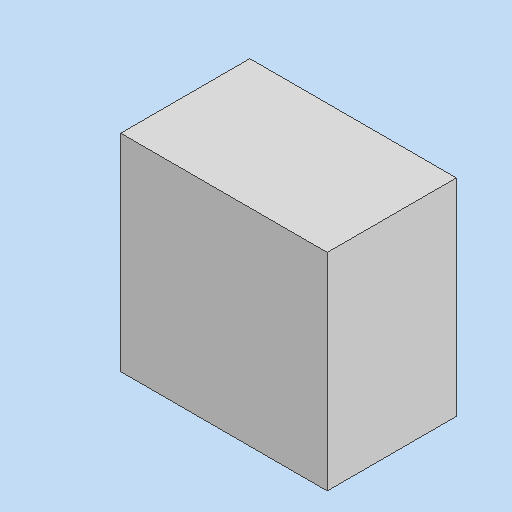
# Autodesk Inventor part: NurdShooterStandin
Saved by Autodesk Inventor 2024.2 (Build 282272000, 272)
## iProperties
Created: 2024-02-06
Part Number: NurdShooterStandin
Material: Generic
Document SubType Name: Modeling
Designer: webbgamers
Density: 1 g/cm^3
Appearance: Default
Author: webbgamers
Autodesk Inventor part; units mm, degrees
ref_plane "YZ Plane" through (0, 0, 0) normal (1, 0, 0) x (0, 1, 0)
ref_plane "XZ Plane" through (0, 0, 0) normal (0, 1, 0) x (-1, 0, 0)
ref_plane "XY Plane" through (0, 0, 0) normal (0, 0, 1) x (1, 0, 0)
ref_plane "Work Plane1" through (1.9437, -39.5479, 0) normal (0, 0, 1) x (1, 0, 0)
sketch "Sketch1" plane through (1.9437, -39.5479, 0) normal (0, 0, 1) x (1, 0, 0)
  line L0 (516.6956, 198.2733) -> (110.2956, 198.2733)
  line L1 (110.2956, 198.2733) -> (110.2956, -208.1267)
  line L2 (110.2956, -208.1267) -> (516.6956, -208.1267)
  line L3 (516.6956, -208.1267) -> (516.6956, 198.2733)
  point P0 (-1.9437, 39.5479)
  dimension "d0" = 406.4
  dimension "d1" = 406.4
  constraints: 8 end point, 2 parallel, 1 horizontal, 1 perpendicular
  measures "d0" distance of L1.end L2.end
  measures "d1" distance of L0.end L1.end
extrude "Extrusion1" add sketch "Sketch1" along normal blind 254
body "Solid1"
